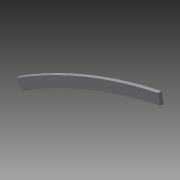
# Autodesk Inventor part: nd-8
Saved by Autodesk Inventor 2015 (Build 190159000, 159)
## iProperties
Created: 2014-07-02
Part Number: nd-8
Material: Generic
Document SubType Name: Modeling
Designer: peter
Density: 1 g/cm^3
Appearance: Default
Author: peter
Autodesk Inventor part; units mm, degrees
ref_plane "YZ Plane" through (0, 0, 0) normal (1, 0, 0) x (0, 1, 0)
ref_plane "XZ Plane" through (0, 0, 0) normal (0, 1, 0) x (-1, 0, 0)
ref_plane "XY Plane" through (0, 0, 0) normal (0, 0, 1) x (1, 0, 0)
sketch "Sketch1" plane through (0, 0, 0) normal (0, 0, 1) x (1, 0, 0)
  arc A0 (781.9975, 368.9913) -> (0.0178, 48.3373) centre (1304.5744, -2019.2535) ccw
  arc A1 (795.1768, 371.837) -> (781.9975, 368.9913) centre (1304.5744, -2019.2535) ccw
  line L0 (795.1768, 371.837) -> (807.0848, 315.9414)
  arc A2 (807.0848, 315.9414) -> (161.9971, 77.2074) centre (1304.5744, -2019.2541) ccw
  arc A3 (161.9971, 77.2074) -> (30.5761, 0.0433) centre (1304.5744, -2019.2541) ccw
  line L1 (30.5761, 0.0433) -> (0.0178, 48.3373)
  point P0 (0, 0)
  constraints: 9 point on circle, 4 centre point, 4 end point
extrude "Extrusion1" add sketch "Sketch1" along normal blind 19.05
body "Solid1"
